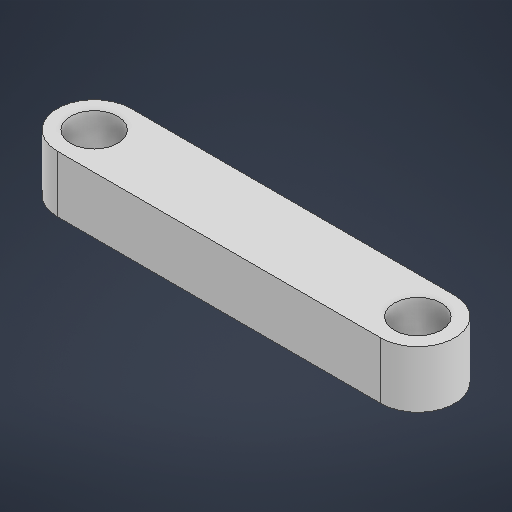
# Autodesk Inventor part: innerBar
Saved by Autodesk Inventor 2026.2 (Build 302298000, 298)
## iProperties
Created: 2026-04-07
Part Number: innerBar
Material: Generic
Document SubType Name: Modeling
Designer: Brian Wang
Density: 1 g/cm^3
Appearance: Default
Author: Brian Wang
Autodesk Inventor part; units mm, degrees
ref_plane "YZ Plane" through (0, 0, 0) normal (1, 0, 0) x (0, 1, 0)
ref_plane "XZ Plane" through (0, 0, 0) normal (0, 1, 0) x (-1, 0, 0)
ref_plane "XY Plane" through (0, 0, 0) normal (0, 0, 1) x (1, 0, 0)
sketch "Sketch1" plane through (0, 0, 0) normal (0, 1, 0) x (-1, 0, 0)
  circle A0 centre (27.2044, 12.7622) radius 2.075
  arc A1 (27.2044, 9.5122) -> (27.2044, 16.0122) centre (27.2044, 12.7622) ccw
  circle A2 centre (-1.2956, 12.7622) radius 2.075
  arc A3 (-1.2956, 16.0122) -> (-1.2956, 9.5122) centre (-1.2956, 12.7622) ccw
  line L0 (27.2044, 16.0122) -> (-1.2956, 16.0122)
  line L1 (27.2044, 9.5122) -> (-1.2956, 9.5122)
  point P0 (0, 0)
  dimension "d1" = 4.15
  dimension "d4" = 4.15
  constraints: 4 centre point, 4 end point, 4 point on circle, 2 coincident, 2 tangent, 1 horizontal alignment
  measures "d1" diameter of A0
  measures "d4" diameter of A2
extrude "Extrusion1" add sketch "Sketch1" along normal blind 5
body "Solid1"
